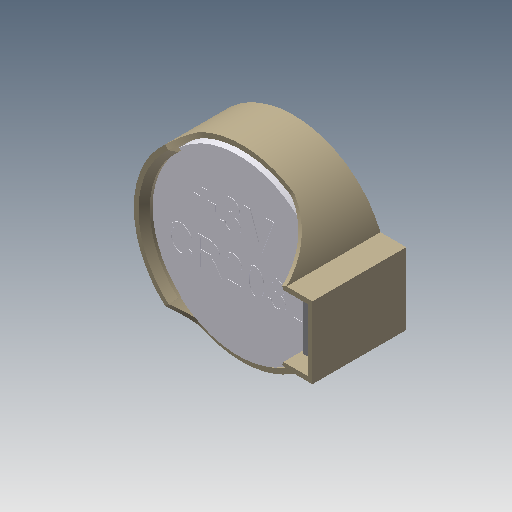
# Autodesk Inventor part: config - battery
Saved by Autodesk Inventor 2020 (Build 240152000, 152)
## iProperties
Created: 2005-12-06
Part Number: config - battery
Document SubType Name: Modeling
Designer: Simon.Ng@autodesk.com
Stock Number: config - battery
Density: 1 g/cm^3
Material: Generic
Mass: 1.86777 g
Surface Area: 20.1612 cm^2
Volume: 1.86777 cm^3
Appearance: Beige
Company: Autodesk Asia Pte. Ltd.
Title: PC Demo
Author: Simon.Ng@autodesk.com
Autodesk Inventor part; units mm, degrees
ref_plane "YZ Plane" through (0, 0, 0) normal (1, 0, 0) x (0, 1, 0)
ref_plane "XZ Plane" through (0, 0, 0) normal (0, 1, 0) x (-1, 0, 0)
sketch "Sketch1" plane through (0, 0, 0) normal (0, 0, 1) x (1, 0, 0)
  line L0 (0, 16) -> (0, -12) projected
  line L1 (-12, 0) -> (16, 0) projected
  circle A0 centre (0, 0) radius 10
  dimension "d0" = 20
  constraints: 2 point on line, 1 centre point
  measures "d0" diameter of A0
extrude "Extrusion1" add sketch "Sketch1" along normal blind 10
shell "Shell1" thickness 0.5 removed faces 1 at (-1.182, 3.1167, 10)
ref_plane "Work Plane1" through (0, 15, 0) normal (0, 1, 0) x (-1, 0, 0)
sketch "Sketch2" plane through (0, 15, 0) normal (0, 1, 0) x (-1, 0, 0)
  line L0 (0, -1) -> (0, 13) projected
  line L1 (-10, 10) -> (10, 10) projected
  arc A0 (-11.7919, 10) -> (-5.8969, 5.5) centre (-3.3291, 14.975) ccw
  line L2 (-5.8969, 5.5) -> (4.6792, 5.5)
  arc A1 (4.6792, 5.5) -> (9.3583, 10) centre (2.2728, 12.6849) ccw
  line L3 (-10, 0) -> (10, 0) projected
  line L4 (-11.7919, 10) -> (9.3583, 10)
  dimension "d5" = 5.5
  constraints: 4 end point, 4 point on circle, 2 centre point, 2 point on line, 1 collinear, 1 parallel
  measures "d5" distance between parallel lines of L3 L2
emboss "Emboss1" sketch "Sketch2" operation cut depth 0.5 direction (0, 1, 0) wrap yes faces at (9.8705, -1.6041, 6.6667)
fillet "Fillet1" radius 2 2 edges at (5.422, 8.1033, 5.5) (-4.3975, 8.702, 5.5)
mirror "Mirror1" about plane through (0, 0, 0) normal (0, 1, 0) of "Emboss1", "Fillet1"
sketch "Sketch3" plane through (0, 0, 10) normal (0, 0, 1) x (1, 0, 0)
  line L0 (-13.5909, 11.9498) -> (-5.9559, 11.9498)
  line L1 (-5.9559, 11.9498) -> (-5.9559, -17.7363)
  line L2 (-5.9559, -17.7363) -> (-13.5909, -17.7363)
  line L3 (-13.5909, -17.7363) -> (-13.5909, 11.9498)
  constraints: 8 end point, 2 parallel, 1 horizontal, 1 perpendicular
extrude "Extrusion2" cut sketch "Sketch3" against normal blind 3
sketch "Sketch4" plane through (0, 0, 10) normal (0, 0, 1) x (1, 0, 0)
  arc A0 (9.243, -3.8167) -> (9.243, 3.8167) centre (0, 0) ccw projected
  line L0 (9.243, 3.8167) -> (12, 3.8167)
  line L1 (12, 3.8167) -> (12, -3.8167)
  line L2 (12, -3.8167) -> (9.243, -3.8167)
  line L3 (9.243, -3.8167) -> (9.243, 3.8167)
  dimension "d11" = 12
  constraints: 8 end point, 2 parallel, 1 horizontal, 1 perpendicular
  measures "d11" distance from line of A0.centre L1
extrude "Extrusion3" add sketch "Sketch4" against normal up to surface (10 mm away)
sketch "Sketch5" plane through (0, 0, 10) normal (0, 0, 1) x (1, 0, 0)
  line L0 (9.243, -3.8167) -> (12, -3.8167) projected
  line L1 (12, -3.8167) -> (12, 3.8167) projected
  line L2 (12, 3.8167) -> (9.243, 3.8167) projected
  line L3 (7.6156, 3.3167) -> (11.5, 3.3167)
  line L4 (11.5, 3.3167) -> (11.5, -3.3167)
  line L5 (11.5, -3.3167) -> (7.6156, -3.3167)
  line L6 (7.6156, -3.3167) -> (7.6156, 3.3167)
  dimension "d14" = 0.5
  dimension "d15" = 0.5
  dimension "d16" = 0.5
  constraints: 8 end point, 2 parallel, 1 horizontal, 1 perpendicular
  measures "d14" distance between parallel lines of L1 L4
  measures "d15" distance between parallel lines of L2 L3
extrude "Extrusion4" cut sketch "Sketch5" against normal up to surface (9.5 mm away)
sketch "Sketch6" plane through (0, 0, 0) normal (0, 1, 0) x (-1, 0, 0)
  line L0 (9.5, 0.5) -> (9.5, 7) projected
  line L1 (9.5, 7) -> (9, 6.3)
  line L2 (9, 6.3) -> (9, 6)
  line L3 (9, 6) -> (9.5, 6)
  line L4 (9.5, 6) -> (9.5, 7)
  dimension "d19" = 1
  dimension "d20" = 0.3
  dimension "d21" = 0.5
  constraints: 8 end point, 1 collinear, 1 parallel, 1 perpendicular, 1 point on line
  measures "d19" distance of L3.end L0.end
  measures "d20" distance of L1.end L2.end
  measures "d21" distance between parallel lines of L0 L2
sketch "Sketch7" plane through (0, 0, 7) normal (0, 0, 1) x (1, 0, 0)
  arc A0 (-6.3227, 7.0903) -> (-6.3227, -7.0903) centre (0, 0) ccw projected
sweep "Sweep1" add profiles "Sketch6" path "Sketch7"
sketch "Sketch8" plane through (8.9022, -3.3167, 0.5) normal (0, 0, 1) x (1, 0, 0)
  arc A0 (0, 6.6335) -> (0, 0) centre (-8.9022, 3.3167) ccw projected
  circle A1 centre (-8.9022, 3.3167) radius 9.25
  dimension "d23" = 18.5
  constraints: 1 centre point, 1 coincident
  measures "d23" diameter of A1
extrude "Extrusion5" add sketch "Sketch8" along normal blind 5.4
sketch "Sketch9" plane through (8.9022, -3.3167, 0.5) normal (0, 0, 1) x (1, 0, 0)
  line L0 (-21.1022, 3.3167) -> (9.6978, 3.3167) projected
  line L1 (0.5978, 6.3167) -> (1.0978, 6.3167)
  line L2 (1.0978, 6.3167) -> (1.0978, 0.3167)
  line L3 (1.0978, 0.3167) -> (0.5978, 0.3167)
  line L4 (0.5978, 0.3167) -> (0.5978, 6.3167)
  line L5 (-8.9022, 25.3419) -> (-8.9022, -13.2021) projected
  dimension "d26" = 9.5
  dimension "d27" = 0.5
  dimension "d28" = 6
  constraints: 8 end point, 2 parallel, 1 horizontal, 1 perpendicular, 1 other
  measures "d26" distance between parallel lines of L4 L5
  measures "d27" distance of L2.end L3.end
  measures "d28" distance of L1.end L2.end
extrude "Extrusion6" add sketch "Sketch9" along normal blind 8
sketch "Sketch10" plane through (0, 0, 0) normal (0, 1, 0) x (-1, 0, 0)
  line L0 (-9.5, 0.5) -> (-9.5, 8.5) projected
  line L1 (-9.5, 8.5) -> (-8, 6)
  line L2 (-8, 6) -> (-9.5, 6)
  line L3 (-9.25, 5.9) -> (9.25, 5.9) projected
  line L4 (-10, 0.5) -> (-10, 8.5) projected
  dimension "d31" = 0.1
  dimension "d32" = 2
  constraints: 4 end point, 1 perpendicular, 1 point on line
  measures "d31" distance between parallel lines of L2 L3
  measures "d32" distance from line of L4 L1.end
extrude "Extrusion7" add sketch "Sketch10" along normal mid plane 6
sketch "Sketch11" plane through (0, 0, 5.9) normal (0, 0, 1) x (1, 0, 0)
  line L0 (-12.2, 0) -> (18.6, 0) projected
  line L1 (9.5, 3) -> (8, 3) projected
  line L2 (8, -3) -> (9.5, -3) projected
  line L3 (9.5, 3) -> (8, 3) projected
  line L4 (8, -3) -> (8, 3) projected
  line L5 (8, -3) -> (9.5, -3) projected
  line L6 (9.5, -3) -> (9.5, 3) projected
  line L7 (8, 2.5) -> (9.5, 2.5)
  line L8 (9.5, 2.5) -> (9.5, -2.5)
  line L9 (9.5, -2.5) -> (8, -2.5)
  line L10 (8, -2.5) -> (8, 2.5)
  dimension "d35" = 0.5
  dimension "d36" = 0.5
  constraints: 8 end point, 2 parallel, 2 point on line, 1 horizontal, 1 perpendicular
  measures "d35" distance between parallel lines of L1 L7
  measures "d36" distance between parallel lines of L2 L9
extrude "Extrusion8" cut sketch "Sketch11" along normal through all contours L4 L7 L6 L0 | L0 L6 L9 L4
sketch "Sketch12" plane through (0, 0, 5.9) normal (0, 0, 1) x (1, 0, 0)
  line L0 (-5.0186, 4.9757) -> (3.8168, 4.9757) construction
  line L1 (3.8168, 4.9757) -> (3.8168, 1.4037) construction
  line L2 (3.8168, 1.4037) -> (-5.0186, 1.4037) construction
  line L3 (-5.0186, 1.4037) -> (-5.0186, 4.9757) construction
  line L4 (-7.7209, 0) -> (10.2166, 0) construction
  line L5 (10.2166, 0) -> (10.2166, -3.62) construction
  line L6 (10.2166, -3.62) -> (-7.7209, -3.62) construction
  line L7 (-7.7209, -3.62) -> (-7.7209, 0) construction
  line L8 (-3.8981, 1.9665) -> (-3.8981, 2.8735)
  line L9 (-3.8981, 2.8735) -> (-4.8158, 2.8735)
  line L10 (-4.8158, 2.8735) -> (-4.8158, 3.5005)
  line L11 (-4.8158, 3.5005) -> (-3.8981, 3.5005)
  line L12 (-3.8981, 3.5005) -> (-3.8981, 4.4075)
  line L13 (-3.8981, 4.4075) -> (-3.2872, 4.4075)
  line L14 (-3.2872, 4.4075) -> (-3.2872, 3.5005)
  line L15 (-3.2872, 3.5005) -> (-2.3669, 3.5005)
  line L16 (-2.3669, 3.5005) -> (-2.3669, 2.8735)
  line L17 (-2.3669, 2.8735) -> (-3.2872, 2.8735)
  line L18 (-3.2872, 2.8735) -> (-3.2872, 1.9665)
  line L19 (-3.2872, 1.9665) -> (-3.8981, 1.9665)
  line L20 (-1.9801, 2.3934) -> (-1.3318, 2.4734)
  spline S0 degree 3 poles (-1.3318, 2.4734) (-1.2998, 2.2253) (-1.0277, 1.9612) (-0.8356, 1.9612) knots 0 0 0 0 1 1 1 1
  spline S1 degree 3 poles (-0.8356, 1.9612) (-0.6276, 1.9612) (-0.3448, 2.276) (-0.3448, 2.5428) knots 0 0 0 0 1 1 1 1
  spline S2 degree 3 poles (-0.3448, 2.5428) (-0.3448, 2.7962) (-0.6142, 3.0923) (-0.809, 3.0923) knots 0 0 0 0 1 1 1 1
  spline S3 degree 2 poles (-0.809, 3.0923) (-0.937, 3.0923) (-1.1158, 3.0416) knots 0 0 0 1 1 1
  line L21 (-1.1158, 3.0416) -> (-1.0411, 3.5885)
  spline S4 degree 3 poles (-1.0411, 3.5885) (-0.769, 3.5805) (-0.4835, 3.8312) (-0.4835, 4.0393) knots 0 0 0 0 1 1 1 1
  spline S5 degree 3 poles (-0.4835, 4.0393) (-0.4835, 4.2154) (-0.6943, 4.4235) (-0.8677, 4.4235) knots 0 0 0 0 1 1 1 1
  spline S6 degree 3 poles (-0.8677, 4.4235) (-1.0411, 4.4235) (-1.2838, 4.186) (-1.3105, 3.9566) knots 0 0 0 0 1 1 1 1
  line L22 (-1.3105, 3.9566) -> (-1.9294, 4.0607)
  spline S7 degree 4 poles (-1.9294, 4.0607) (-1.8654, 4.3781) (-1.6039, 4.7596) (-1.1398, 4.9757) (-0.849, 4.9757) knots 0 0 0 0 0 1 1 1 1 1
  spline S8 degree 2 poles (-0.849, 4.9757) (-0.3555, 4.9757) (-0.0567, 4.6609) knots 0 0 0 1 1 1
  spline S9 degree 2 poles (-0.0567, 4.6609) (0.1887, 4.4048) (0.1887, 4.0793) knots 0 0 0 1 1 1
  spline S10 degree 2 poles (0.1887, 4.0793) (0.1887, 3.6205) (-0.3154, 3.3457) knots 0 0 0 1 1 1
  spline S11 degree 3 poles (-0.3154, 3.3457) (-0.014, 3.2817) (0.3435, 2.8309) (0.3435, 2.5134) knots 0 0 0 0 1 1 1 1
  spline S12 degree 3 poles (0.3435, 2.5134) (0.3435, 2.0519) (-0.3288, 1.4037) (-0.8303, 1.4037) knots 0 0 0 0 1 1 1 1
  spline S13 degree 3 poles (-0.8303, 1.4037) (-1.3052, 1.4037) (-1.9294, 1.9505) (-1.9801, 2.3934) knots 0 0 0 0 1 1 1 1
  line L23 (1.8054, 1.4623) -> (0.5542, 4.9623)
  line L24 (0.5542, 4.9623) -> (1.3198, 4.9623)
  line L25 (1.3198, 4.9623) -> (2.2082, 2.372)
  line L26 (2.2082, 2.372) -> (3.0645, 4.9623)
  line L27 (3.0645, 4.9623) -> (3.8141, 4.9623)
  line L28 (3.8141, 4.9623) -> (2.563, 1.4623)
  line L29 (2.563, 1.4623) -> (1.8054, 1.4623)
  line L30 (-5.2582, -1.9985) -> (-4.8604, -2.0991)
  spline S14 degree 3 poles (-4.8604, -2.0991) (-4.9861, -2.5884) (-5.6332, -3.1029) (-6.102, -3.1029) knots 0 0 0 0 1 1 1 1
  spline S15 degree 4 poles (-6.102, -3.1029) (-6.5867, -3.1029) (-7.195, -2.7073) (-7.5128, -1.9596) (-7.5128, -1.5297) knots 0 0 0 0 0 1 1 1 1 1
  spline S16 degree 4 poles (-7.5128, -1.5297) (-7.5128, -1.061) (-7.1538, -0.3613) (-6.493, 0) (-6.0951, 0) knots 0 0 0 0 0 1 1 1 1 1
  spline S17 degree 3 poles (-6.0951, 0) (-5.6447, 0) (-5.0319, -0.4596) (-4.9107, -0.8735) knots 0 0 0 0 1 1 1 1
  line L31 (-4.9107, -0.8735) -> (-5.3017, -0.9672)
  spline S18 degree 3 poles (-5.3017, -0.9672) (-5.4069, -0.6402) (-5.8024, -0.3407) (-6.1043, -0.3407) knots 0 0 0 0 1 1 1 1
  spline S19 degree 4 poles (-6.1043, -0.3407) (-6.4495, -0.3407) (-6.916, -0.6723) (-7.1035, -1.2302) (-7.1035, -1.5274) knots 0 0 0 0 0 1 1 1 1 1
  spline S20 degree 4 poles (-7.1035, -1.5274) (-7.1035, -1.9093) (-6.8794, -2.4809) (-6.4107, -2.7622) (-6.1363, -2.7622) knots 0 0 0 0 0 1 1 1 1 1
  spline S21 degree 3 poles (-6.1363, -2.7622) (-5.8024, -2.7622) (-5.3405, -2.378) (-5.2582, -1.9985) knots 0 0 0 0 1 1 1 1
  line L32 (-4.3642, -3.0526) -> (-4.3642, -0.0526)
  line L33 (-4.3642, -0.0526) -> (-3.0334, -0.0526)
  spline S22 degree 4 poles (-3.0334, -0.0526) (-2.6332, -0.0526) (-2.2148, -0.2149) (-1.9655, -0.6242) (-1.9655, -0.8712) knots 0 0 0 0 0 1 1 1 1 1
  spline S23 degree 3 poles (-1.9655, -0.8712) (-1.9655, -1.1913) (-2.3794, -1.628) (-2.8093, -1.6875) knots 0 0 0 0 1 1 1 1
  spline S24 degree 2 poles (-2.8093, -1.6875) (-2.6538, -1.763) (-2.5715, -1.8361) knots 0 0 0 1 1 1
  spline S25 degree 2 poles (-2.5715, -1.8361) (-2.3977, -1.9962) (-2.2422, -2.2363) knots 0 0 0 1 1 1
  line L34 (-2.2422, -2.2363) -> (-1.7232, -3.0526)
  line L35 (-1.7232, -3.0526) -> (-2.2194, -3.0526)
  line L36 (-2.2194, -3.0526) -> (-2.6172, -2.4284)
  spline S26 degree 4 poles (-2.6172, -2.4284) (-2.791, -2.1585) (-3.0151, -1.8727) (-3.1934, -1.7561) (-3.2849, -1.7332) knots 0 0 0 0 0 1 1 1 1 1
  spline S27 degree 2 poles (-3.2849, -1.7332) (-3.3535, -1.7195) (-3.5067, -1.7195) knots 0 0 0 1 1 1
  line L37 (-3.5067, -1.7195) -> (-3.9663, -1.7195)
  line L38 (-3.9663, -1.7195) -> (-3.9663, -3.0526)
  line L39 (-3.9663, -3.0526) -> (-4.3642, -3.0526)
  line L40 (-3.9663, -1.3765) -> (-3.1134, -1.3765)
  spline S28 degree 4 poles (-3.1134, -1.3765) (-2.8413, -1.3765) (-2.5349, -1.2645) (-2.3748, -1.0152) (-2.3748, -0.8712) knots 0 0 0 0 0 1 1 1 1 1
  spline S29 degree 3 poles (-2.3748, -0.8712) (-2.3748, -0.6585) (-2.6835, -0.3841) (-3.0174, -0.3841) knots 0 0 0 0 1 1 1 1
  line L41 (-3.0174, -0.3841) -> (-3.9663, -0.3841)
  line L42 (-3.9663, -0.3841) -> (-3.9663, -1.3765)
  line L43 (0.4422, -2.6982) -> (0.4422, -3.0526)
  line L44 (0.4422, -3.0526) -> (-1.5402, -3.0526)
  spline S30 degree 2 poles (-1.5402, -3.0526) (-1.5448, -2.92) (-1.4968, -2.7965) knots 0 0 0 1 1 1
  spline S31 degree 3 poles (-1.4968, -2.7965) (-1.4213, -2.593) (-1.0875, -2.202) (-0.772, -1.9436) knots 0 0 0 0 1 1 1 1
  spline S32 degree 3 poles (-0.772, -1.9436) (-0.2849, -1.5412) (0.0581, -1.0747) (0.0581, -0.8643) knots 0 0 0 0 1 1 1 1
  spline S33 degree 3 poles (0.0581, -0.8643) (0.0581, -0.6448) (-0.2552, -0.3453) (-0.5067, -0.3453) knots 0 0 0 0 1 1 1 1
  spline S34 degree 3 poles (-0.5067, -0.3453) (-0.772, -0.3453) (-1.0898, -0.6654) (-1.0921, -0.9466) knots 0 0 0 0 1 1 1 1
  line L45 (-1.0921, -0.9466) -> (-1.4716, -0.9078)
  spline S35 degree 3 poles (-1.4716, -0.9078) (-1.4328, -0.4848) (-0.9252, -0.0412) (-0.4976, -0.0412) knots 0 0 0 0 1 1 1 1
  spline S36 degree 3 poles (-0.4976, -0.0412) (-0.0654, -0.0412) (0.4377, -0.5191) (0.4377, -0.8735) knots 0 0 0 0 1 1 1 1
  spline S37 degree 4 poles (0.4377, -0.8735) (0.4377, -1.0541) (0.2913, -1.4017) (-0.0517, -1.7858) (-0.4473, -2.122) knots 0 0 0 0 0 1 1 1 1 1
  spline S38 degree 3 poles (-0.4473, -2.122) (-0.7788, -2.3986) (-0.9663, -2.5976) (-1.028, -2.6982) knots 0 0 0 0 1 1 1 1
  line L46 (-1.028, -2.6982) -> (0.4422, -2.6982)
  spline S39 degree 4 poles (0.8378, -1.5732) (0.8378, -1.0404) (1.0573, -0.391) (1.4872, -0.0412) (1.8165, -0.0412) knots 0 0 0 0 0 1 1 1 1 1
  spline S40 degree 5 poles (1.8165, -0.0412) (2.0566, -0.0412) (2.4224, -0.2355) (2.6579, -0.6014) (2.7928, -1.1273) (2.7928, -1.5732) knots 0 0 0 0 0 0 1 1 1 1 1 1
  spline S41 degree 4 poles (2.7928, -1.5732) (2.7928, -2.1014) (2.5756, -2.7508) (2.1434, -3.1029) (1.8165, -3.1029) knots 0 0 0 0 0 1 1 1 1 1
  spline S42 degree 2 poles (1.8165, -3.1029) (1.382, -3.1029) (1.1351, -2.7942) knots 0 0 0 1 1 1
  spline S43 degree 2 poles (1.1351, -2.7942) (0.8378, -2.4169) (0.8378, -1.5732) knots 0 0 0 1 1 1
  spline S44 degree 3 poles (1.2174, -1.5732) (1.2174, -2.314) (1.5627, -2.8011) (1.8165, -2.8011) knots 0 0 0 0 1 1 1 1
  spline S45 degree 3 poles (1.8165, -2.8011) (2.068, -2.8011) (2.4133, -2.3117) (2.4133, -1.5732) knots 0 0 0 0 1 1 1 1
  spline S46 degree 3 poles (2.4133, -1.5732) (2.4133, -0.8323) (2.068, -0.3453) (1.8119, -0.3453) knots 0 0 0 0 1 1 1 1
  spline S47 degree 2 poles (1.8119, -0.3453) (1.5581, -0.3453) (1.4072, -0.5602) knots 0 0 0 1 1 1
  spline S48 degree 2 poles (1.4072, -0.5602) (1.2174, -0.8346) (1.2174, -1.5732) knots 0 0 0 1 1 1
  line L47 (3.1701, -2.2569) -> (3.5383, -2.2088)
  spline S49 degree 3 poles (3.5383, -2.2088) (3.6023, -2.5221) (3.9064, -2.7988) (4.1259, -2.7988) knots 0 0 0 0 1 1 1 1
  spline S50 degree 3 poles (4.1259, -2.7988) (4.3866, -2.7988) (4.7433, -2.4375) (4.7433, -2.1723) knots 0 0 0 0 1 1 1 1
  spline S51 degree 3 poles (4.7433, -2.1723) (4.7433, -1.9184) (4.4117, -1.5892) (4.1556, -1.5892) knots 0 0 0 0 1 1 1 1
  spline S52 degree 2 poles (4.1556, -1.5892) (4.0527, -1.5892) (3.8973, -1.6303) knots 0 0 0 1 1 1
  line L48 (3.8973, -1.6303) -> (3.9361, -1.3079)
  spline S53 degree 2 poles (3.9361, -1.3079) (3.975, -1.3125) (3.9956, -1.3125) knots 0 0 0 1 1 1
  spline S54 degree 3 poles (3.9956, -1.3125) (4.2311, -1.3125) (4.6084, -1.0655) (4.6084, -0.8117) knots 0 0 0 0 1 1 1 1
  spline S55 degree 3 poles (4.6084, -0.8117) (4.6084, -0.6082) (4.334, -0.343) (4.1168, -0.343) knots 0 0 0 0 1 1 1 1
  spline S56 degree 3 poles (4.1168, -0.343) (3.9018, -0.343) (3.616, -0.6128) (3.5748, -0.8849) knots 0 0 0 0 1 1 1 1
  line L49 (3.5748, -0.8849) -> (3.2067, -0.8186)
  spline S57 degree 3 poles (3.2067, -0.8186) (3.2753, -0.4482) (3.7532, -0.0412) (4.1099, -0.0412) knots 0 0 0 0 1 1 1 1
  spline S58 degree 4 poles (4.1099, -0.0412) (4.3546, -0.0412) (4.7684, -0.2515) (4.988, -0.6151) (4.988, -0.8186) knots 0 0 0 0 0 1 1 1 1 1
  spline S59 degree 3 poles (4.988, -0.8186) (4.988, -1.013) (4.7799, -1.3331) (4.5741, -1.4268) knots 0 0 0 0 1 1 1 1
  spline S60 degree 3 poles (4.5741, -1.4268) (4.8416, -1.4886) (5.1343, -1.875) (5.1343, -2.1654) knots 0 0 0 0 1 1 1 1
  spline S61 degree 3 poles (5.1343, -2.1654) (5.1343, -2.5564) (4.5604, -3.1029) (4.1236, -3.1029) knots 0 0 0 0 1 1 1 1
  spline S62 degree 3 poles (4.1236, -3.1029) (3.728, -3.1029) (3.2067, -2.6319) (3.1701, -2.2569) knots 0 0 0 0 1 1 1 1
  line L50 (7.4323, -2.6982) -> (7.4323, -3.0526)
  line L51 (7.4323, -3.0526) -> (5.4498, -3.0526)
  spline S63 degree 2 poles (5.4498, -3.0526) (5.4453, -2.92) (5.4933, -2.7965) knots 0 0 0 1 1 1
  spline S64 degree 3 poles (5.4933, -2.7965) (5.5688, -2.593) (5.9026, -2.202) (6.2181, -1.9436) knots 0 0 0 0 1 1 1 1
  spline S65 degree 3 poles (6.2181, -1.9436) (6.7052, -1.5412) (7.0482, -1.0747) (7.0482, -0.8643) knots 0 0 0 0 1 1 1 1
  spline S66 degree 3 poles (7.0482, -0.8643) (7.0482, -0.6448) (6.7349, -0.3453) (6.4834, -0.3453) knots 0 0 0 0 1 1 1 1
  spline S67 degree 3 poles (6.4834, -0.3453) (6.2181, -0.3453) (5.9003, -0.6654) (5.898, -0.9466) knots 0 0 0 0 1 1 1 1
  line L52 (5.898, -0.9466) -> (5.5184, -0.9078)
  spline S68 degree 3 poles (5.5184, -0.9078) (5.5573, -0.4848) (6.0649, -0.0412) (6.4925, -0.0412) knots 0 0 0 0 1 1 1 1
  spline S69 degree 3 poles (6.4925, -0.0412) (6.9247, -0.0412) (7.4277, -0.5191) (7.4277, -0.8735) knots 0 0 0 0 1 1 1 1
  spline S70 degree 4 poles (7.4277, -0.8735) (7.4277, -1.0541) (7.2814, -1.4017) (6.9384, -1.7858) (6.5428, -2.122) knots 0 0 0 0 0 1 1 1 1 1
  spline S71 degree 3 poles (6.5428, -2.122) (6.2113, -2.3986) (6.0238, -2.5976) (5.962, -2.6982) knots 0 0 0 0 1 1 1 1
  line L53 (5.962, -2.6982) -> (7.4323, -2.6982)
  constraints: 4 other
extrude "Extrusion9" add sketch "Sketch12" along normal blind 0.05
equation "\"d36\" = d35"
body "Solid1"
